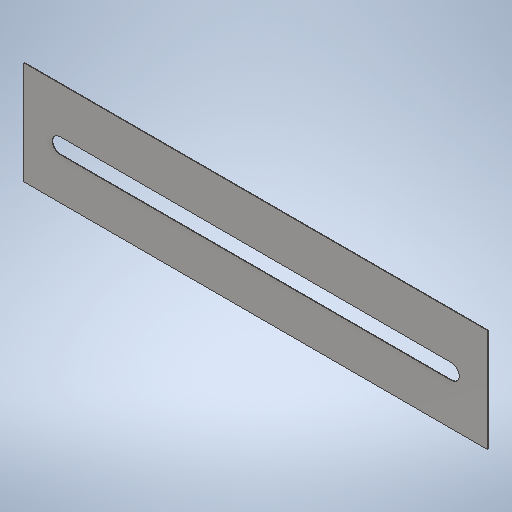
# Autodesk Inventor part: project slit
Saved by Autodesk Inventor 2025.2 (Build 292293000, 293)
## iProperties
Created: 2025-02-04
Part Number: project slit
Material: Steel, Galvanized
Document SubType Name: Sheet Metal
Designer: nandu
Density: 7.85 g/cm^3
Sheet Metal Rule: Default_mm
Appearance: Galvanized
Author: nandu
Autodesk Inventor part; units mm, degrees
ref_plane "YZ Plane" through (0, 0, 0) normal (1, 0, 0) x (0, 1, 0)
ref_plane "XZ Plane" through (0, 0, 0) normal (0, 1, 0) x (-1, 0, 0)
ref_plane "XY Plane" through (0, 0, 0) normal (0, 0, 1) x (1, 0, 0)
sketch "Sketch1" plane through (0, 0, 0) normal (0, 0, 1) x (1, 0, 0)
  line L0 (0, 0) -> (450, 0)
  line L1 (450, 0) -> (450, 100)
  line L2 (450, 100) -> (0, 100)
  line L3 (0, 100) -> (0, 0)
  line L4 (35, 40.5) -> (415, 40.5)
  line L5 (415, 40.5) -> (415, 55.5)
  line L6 (415, 55.5) -> (35, 55.5)
  line L7 (35, 55.5) -> (35, 40.5)
  circle A0 centre (35, 48) radius 7.5
  circle A1 centre (415, 48) radius 7.5
  point P0 (35, 40.5)
  point P1 (35, 55.5)
  dimension "d0" = 450
  dimension "d1" = 100
  dimension "d2" = 380
  dimension "d3" = 15
  dimension "d4" = 15
  dimension "d5" = 15
  dimension "d8" = 35
  dimension "d9" = 52
  constraints: 16 end point, 4 parallel, 2 centre point, 2 horizontal, 2 midpoint, 2 perpendicular
  measures "d0" distance of L2.end L1.end
  measures "d1" distance of L1.end L0.end
  measures "d2" distance of L6.end L5.end
  measures "d3" distance of L5.end L4.end
  measures "d4" diameter of A0
  measures "d5" diameter of A1
  measures "d8" distance between parallel lines of L3 L7
  measures "d9" distance from line of L2 A1.centre
extrude "Extrusion1" add sketch "Sketch1" along normal blind 0.602
equation "\"BendRadius\" = Thickness"
equation "\"BendReliefWidth\" = Thickness"
equation "\"BendReliefDepth\" = 0.5 * Thickness"
equation "\"CornerReliefSize\" = 4 * Thickness"
equation "\"MinimumRemnant\" = 2 * Thickness"
equation "\"TransitionRadius\" = BendRadius"
equation "\"JacobiRadiusSize\" = BendRadius"
equation "\"GapSize\" = Thickness"
equation "\"Thickness\" = 0.602"
body "Solid1"
